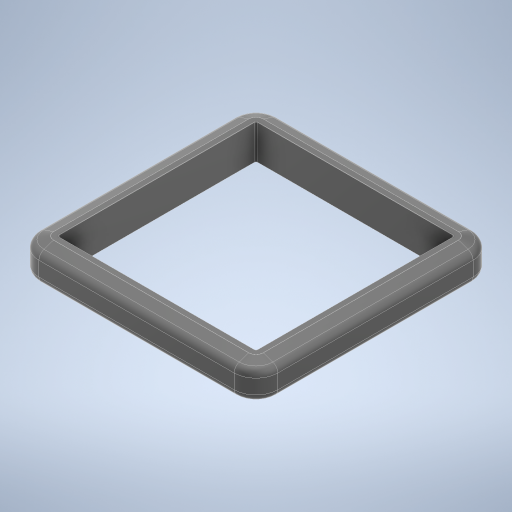
# Autodesk Inventor part: Cover
Saved by Autodesk Inventor 2023 (Build 270158000, 158)
## iProperties
Created: 2023-11-22
Part Number: Cover
Material: Generic
Document SubType Name: Modeling
Designer: adamarnold
Density: 1 g/cm^3
Appearance: Smooth - Black
Author: adamarnold
Autodesk Inventor part; units mm, degrees
ref_plane "XZ Plane" through (0, 0, 0) normal (0, 1, 0) x (-1, 0, 0)
ref_plane "XY Plane" through (0, 0, 0) normal (0, 0, 1) x (1, 0, 0)
sketch "Sketch1" plane through (0, 0, 0) normal (0, 1, 0) x (-1, 0, 0)
  line L0 (50.8, 0) -> (733.425, 0)
  line L1 (784.225, -50.8) -> (784.225, -733.425)
  line L2 (733.425, -784.225) -> (50.8, -784.225)
  line L3 (0, -733.425) -> (0, -50.8)
  arc A0 (784.225, -50.8) -> (733.425, 0) centre (733.425, -50.8) ccw
  arc A1 (733.425, -784.225) -> (784.225, -733.425) centre (733.425, -733.425) ccw
  arc A2 (0, -733.425) -> (50.8, -784.225) centre (50.8, -733.425) ccw
  arc A3 (50.8, 0) -> (0, -50.8) centre (50.8, -50.8) ccw
  point P0 (0, 0)
  point P1 (784.225, -784.225)
  point P2 (784.225, 0)
  point P3 (0, -784.225)
  dimension "d0" = 784.225
  dimension "d1" = 784.225
  dimension "d12" = 50.8
  constraints: 8 end point, 8 point on circle, 8 point on line, 8 tangent, 4 centre point, 3 equal radius, 2 parallel, 1 horizontal, 1 perpendicular
  measures "d0" distance of point (784.225, -784.225) point (0, -784.225)
  measures "d1" distance of point (784.225, 0) point (784.225, -784.225)
  measures "d12" radius of A0
ref_plane "Work Plane1" through (-392.1125, 0, 0) normal (1, 0, 0) x (0, 1, 0)
sketch "Sketch2" plane through (-392.1125, 0, 0) normal (1, 0, 0) x (0, 1, 0)
  line L0 (0, 0) -> (0, -45.085)
  line L1 (0, -45.085) -> (60.198, -45.085)
  line L2 (0, 0) -> (25.4, 0)
  line L3 (60.96, -44.323) -> (60.96, -25.647)
  line L4 (60.882, -25.1657) -> (49.8011, 8.1226)
  arc A0 (60.198, -45.085) -> (60.96, -44.323) centre (60.198, -44.323) ccw
  arc A1 (60.96, -25.647) -> (60.882, -25.1657) centre (59.436, -25.647) ccw
  line L5 (0, 0) -> (0, 25.7175)
  line L6 (0, 25.7175) -> (25.4, 25.7175)
  arc A2 (49.8011, 8.1226) -> (25.4, 25.7175) centre (25.4, 0) ccw
  line L7 (0, -45.085) -> (-60.198, -45.085)
  line L8 (-60.96, -44.323) -> (-60.96, -25.647)
  line L9 (-60.882, -25.1657) -> (-49.8011, 8.1226)
  arc A3 (-60.96, -44.323) -> (-60.198, -45.085) centre (-60.198, -44.323) ccw
  arc A4 (-60.882, -25.1657) -> (-60.96, -25.647) centre (-59.436, -25.647) ccw
  line L10 (0, 25.7175) -> (-25.4, 25.7175)
  arc A5 (-25.4, 25.7175) -> (-49.8011, 8.1226) centre (-25.4, 0) ccw
  point P0 (60.96, -45.085)
  point P1 (60.96, -25.4)
  point P2 (-60.96, -45.085)
  point P3 (-60.96, -25.4)
  dimension "d3" = 45.085
  dimension "d4" = 60.96
  dimension "d5" = 25.4
  dimension "d7" = 19.685
  dimension "d8" = 0.762
  dimension "d9" = 1.524
  dimension "d10" = 25.7175
  dimension "d11" = 25.4
  constraints: 22 end point, 12 point on circle, 11 symmetric about line, 8 point on line, 6 centre point, 6 tangent, 3 vertical, 1 coincident, 1 horizontal, 1 perpendicular, 3 other
  measures "d3" distance of L0.start L0.end
  measures "d4" distance of L0.end point (60.96, -45.085)
  measures "d5" distance of L0.start L2.end
  measures "d7" distance of point (60.96, -45.085) point (60.96, -25.4)
  measures "d8" radius of A0
  measures "d9" radius of A1
  measures "d10" distance of L0.start L5.end
  measures "d11" distance of L5.end L6.end
sweep "Sweep1" add profiles "Sketch2" path "Sketch1" path curves L0 A0 L1 A1 L2 A2 L3 A3
body "Solid1"
